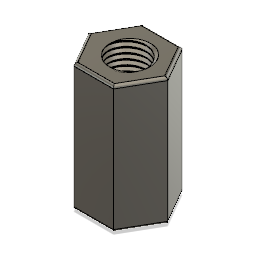
14part (Autodesk Fusion 360 design; units mm, degrees)
Autodesk Fusion 360 part; units mm, degrees
sketch "Sketch1" plane through (0, 0, 0) normal (0, 1, 0) x (1, 0, 0)
  circle A0 centre (0, 0) radius 4
  line L0 (-3.7528, 6.5) -> (-7.5056, 0)
  line L1 (-7.5056, 0) -> (-3.7528, -6.5)
  line L2 (-3.7528, -6.5) -> (3.7528, -6.5)
  line L3 (3.7528, -6.5) -> (7.5056, 0)
  line L4 (7.5056, 0) -> (3.7528, 6.5)
  line L5 (3.7528, 6.5) -> (-3.7528, 6.5)
  dimension "d1" = 8
  dimension "d2" = 6.5
  constraint coincident A0.centre origin
  constraint horizontal L5
  measures "d1" diameter of A0
  measures "d2" distance of A0.centre L5
extrude "Extrude1" add sketch "Sketch1" along normal blind 24
fillet "Fillet1" radius 0.5 12 edges at (0, 0, -6.5) (-5.6292, 0, -3.25) (-5.6292, 0, 3.25) (0, 0, 6.5) (5.6292, 0, 3.25) (5.6292, 0, -3.25) (0, 24, 6.5) (5.6292, 24, 3.25) (5.6292, 24, -3.25) (0, 24, -6.5) (-5.6292, 24, -3.25) (-5.6292, 24, 3.25)
thread "Thread1" "ISO Metric profile 8.0 M8x1 6H" major diameter 8.147 minor diameter 7.035 pitch 1 angle 60 modelled right hand crest width 0.125 on face at (3.995, 16, 0.1994) crest through (3.5175, -0.5625, 0)
